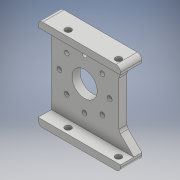
# Autodesk Inventor part: connector_shoulder_jasper
Saved by Autodesk Inventor 2018 (Build 220112000, 112)
## iProperties
Created: 2019-04-16
Part Number: connector_shoulder_jasper
Material: Generic
Document SubType Name: Modeling
Designer: Jasper
Density: 1 g/cm^3
Appearance: Default
Author: Jasper
Autodesk Inventor part; units mm, degrees
ref_plane "YZ Plane" through (0, 0, 0) normal (1, 0, 0) x (0, 1, 0)
ref_plane "XZ Plane" through (0, 0, 0) normal (0, 1, 0) x (-1, 0, 0)
ref_plane "XY Plane" through (0, 0, 0) normal (0, 0, 1) x (1, 0, 0)
sketch "Sketch2" plane through (0, 0, 0) normal (0, 1, 0) x (-1, 0, 0)
  line L0 (18, 20) -> (-18, 20)
  line L1 (-18, 20) -> (-18, -20)
  line L2 (-18, -20) -> (18, -20)
  line L3 (18, -20) -> (18, 20)
  line L4 (18, 20) -> (-18, -20) construction
  line L5 (-18, 20) -> (18, -20) construction
  point P0 (0, 0)
  dimension "d0" = 36
  dimension "d1" = 40
  constraints: 12 end point, 2 midpoint, 2 parallel, 1 horizontal, 1 perpendicular
  measures "d0" distance of L2.end L1.end
  measures "d1" distance of L1.end L0.end
extrude "Extrusion1" add sketch "Sketch2" along normal blind 9.3
sketch "Sketch3" plane through (0, 0, 0) normal (0, -1, 0) x (1, 0, 0)
  line L0 (-18, -17) -> (18, -17)
  line L1 (18, -17) -> (18, 17)
  line L2 (18, 17) -> (-18, 17)
  line L3 (-18, 17) -> (-18, -17)
  line L4 (-18, -17) -> (18, 17) construction
  line L5 (18, -17) -> (-18, 17) construction
  point P0 (0, 0)
  dimension "d4" = 36
  dimension "d5" = 34
  constraints: 12 end point, 2 midpoint, 2 parallel, 1 horizontal, 1 perpendicular
  measures "d4" distance of L2.end L1.end
  measures "d5" distance of L1.end L0.end
extrude "Extrusion2" cut sketch "Sketch3" against normal blind 5.8
sketch "Sketch4" plane through (18, 0, -20) normal (0, 0, -1) x (-1, 0, 0)
  line L0 (0, 0) -> (36, 0) projected
  line L1 (36, 0) -> (36, 9.3) projected
  line L2 (0, 9.3) -> (36, 9.3) projected
  line L3 (0, 0) -> (0, 9.3) projected
  line L4 (36, 0) -> (0, 0) construction
  line L5 (0, 0) -> (0, 2.6) construction
  line L6 (0, 0) -> (0, 9.3) construction
  line L7 (0, 2.6) -> (3.5, 2.6) construction
  line L8 (3.5, 2.6) -> (25.5, 2.6) construction
  circle A0 centre (3.5, 2.6) radius 1.35
  circle A1 centre (25.5, 2.6) radius 1.35
  point P0 (18, 0)
  dimension "d8" = 2.6
  dimension "d9" = 3.5
  dimension "d10" = 22
  dimension "d11" = 180
  dimension "d12" = 2.7
  dimension "d13" = 2.7
  constraints: 6 end point, 2 centre point, 2 coincident, 1 parallel, 1 perpendicular, 1 point on line
  measures "d8" distance of L0.start L5.end
  measures "d9" distance of L5.end L7.end
  measures "d10" distance of L7.end L8.end
  measures "d11" angle of L8 L7
  measures "d12" diameter of A0
  measures "d13" diameter of A1
extrude "Extrusion3" cut sketch "Sketch4" against normal up to surface (40 mm away) contours A0 | A1
sketch "Sketch5" plane through (0, 9.3, 0) normal (0, 1, 0) x (1, 0, 0)
  line L0 (18, -17) -> (18, 17) projected
  line L1 (18, 0) -> (7.5, 0)
  line L2 (18, 0) -> (28.5, 0) construction
  line L3 (7.5, 0) -> (-3.5, 0)
  line L4 (7.5, 0) -> (18.5, 0) construction
  circle A0 centre (7.5, 0) radius 1.025
  circle A1 centre (4.2782, 7.7782) radius 1.025
  circle A2 centre (-3.5, 11) radius 1.025
  circle A3 centre (-11.2782, 7.7782) radius 1.025
  circle A4 centre (-14.5, 0) radius 1.025
  circle A5 centre (-11.2782, -7.7782) radius 1.025
  circle A6 centre (-3.5, -11) radius 1.025
  circle A7 centre (4.2782, -7.7782) radius 1.025
  circle A8 centre (-3.5, 0) radius 5.5
  point P0 (0, 0)
  dimension "d16" = 10.5
  dimension "d17" = 180
  dimension "d18" = 11
  dimension "d19" = 180
  dimension "d20" = 2.05
  dimension "d23" = 360
  dimension "d25" = 11
  constraints: 9 centre point, 8 end point, 4 horizontal, 2 coincident, 2 collinear, 1 midpoint, 17 other
  measures "d16" distance of L1.start L1.end
  measures "d17" angle of L1 L2
  measures "d18" distance of L1.end L3.end
  measures "d19" angle of L3 L4
  measures "d20" diameter of A0
  measures "d25" diameter of A8
extrude "Extrusion4" cut sketch "Sketch5" against normal up to surface (3.5 mm away)
sketch "Sketch6" plane through (0, 9.3, 0) normal (0, 1, 0) x (1, 0, 0)
  line L0 (18, 17) -> (-18, 17) projected
  line L1 (-18, 20) -> (-18, 17) projected
  line L2 (18, 20) -> (-18, 20) projected
  line L3 (18, 17) -> (18, 20) projected
  line L4 (-18, -17) -> (18, -17) projected
  line L5 (18, -20) -> (18, -17) projected
  line L6 (-18, -20) -> (18, -20) projected
  line L7 (-18, -17) -> (-18, -20) projected
  line L8 (18, -17) -> (18, 17) projected
  line L9 (18, 0) -> (11.5, 0)
  line L10 (11.5, 0) -> (11.5, 17)
  line L11 (11.5, 0) -> (11.5, -17)
  line L12 (18, 17) -> (11.5, 10.5)
  line L13 (18, 17) -> (27.1924, 17) construction
  line L14 (-18, -17) -> (18, -17) projected
  line L15 (18, -17) -> (11.5, -10.5)
  line L16 (18, -17) -> (27.1924, -17) construction
  point P0 (0, 0)
  dimension "d28" = 6.5
  dimension "d29" = 135
  dimension "d30" = 135
  constraints: 14 end point, 5 point on line, 2 equal length, 2 horizontal, 1 midpoint, 1 parallel, 1 perpendicular
  measures "d28" distance of L9.start L9.end
  measures "d29" angle of L12 L13
  measures "d30" angle of L16 L15
extrude "Extrusion5" cut sketch "Sketch6" against normal up to surface (3.5 mm away) contours L8 L9 L10 L12 | L8 L15 L11 L9
fillet "Fillet1" radius 2 6 edges at (11.5, 7.55, -10.5) (18, 4.65, -20) (11.5, 7.55, 10.5) (18, 4.65, 20) (-18, 4.65, 20) (-18, 4.65, -20)
body "Solid1"
